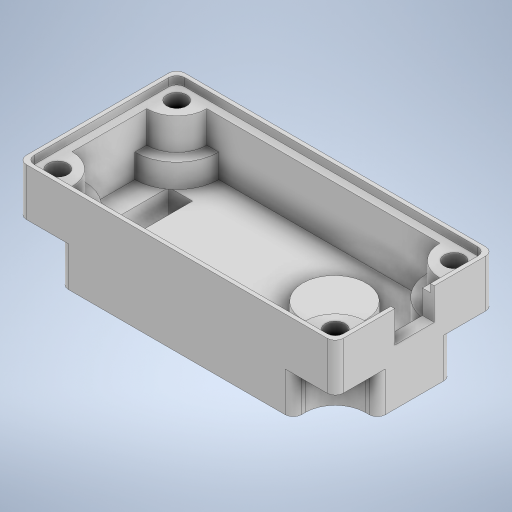
# Autodesk Inventor part: ServoCase
Saved by Autodesk Inventor 2024 (Build 280153000, 153)
## iProperties
Created: 2026-02-12
Part Number: ServoCase
Material: Generic
Document SubType Name: Modeling
Designer: Liam
Density: 1 g/cm^3
Appearance: Default
Author: Liam
Autodesk Inventor part; units mm, degrees
ref_plane "YZ Plane" through (0, 0, 0) normal (1, 0, 0) x (0, 1, 0)
ref_plane "XY Plane" through (0, 0, 0) normal (0, 0, 1) x (1, 0, 0)
sketch "Sketch1" plane through (0, 0, 0) normal (0, 1, 0) x (-1, 0, 0)
  line L0 (20, 10) -> (-20, 10)
  line L1 (-20, 10) -> (-20, -10)
  line L2 (-20, -10) -> (20, -10)
  line L3 (20, -10) -> (20, 10)
  line L4 (20, 10) -> (-20, -10) construction
  line L5 (-20, 10) -> (20, -10) construction
  line L6 (-18.5, 8.5) -> (18.5, 8.5)
  line L7 (18.5, 8.5) -> (18.5, -8.5)
  line L8 (18.5, -8.5) -> (-18.5, -8.5)
  line L9 (-18.5, -8.5) -> (-18.5, 8.5)
  circle A0 centre (17.5, 7.5) radius 1.25
  line L10 (0, 0) -> (18.5, 0) construction
  line L11 (0, 0) -> (0, 0.8088) construction
  line L12 (0, 0.8088) -> (0, 8.5) construction
  circle A1 centre (17.5, -7.5) radius 1.25
  circle A2 centre (-17.5, 7.5) radius 1.25
  circle A3 centre (-17.5, -7.5) radius 1.25
  line L13 (-19.5, 9.5) -> (19.5, 9.5)
  line L14 (19.5, 9.5) -> (19.5, -9.5)
  line L15 (19.5, -9.5) -> (-19.5, -9.5)
  line L16 (-19.5, -9.5) -> (-19.5, 9.5)
  arc A4 (14.7, 8.5) -> (18.5, 4.7) centre (18.5, 8.5) ccw
  arc A5 (18.5, -4.7) -> (14.7, -8.5) centre (18.5, -8.5) ccw
  arc A6 (-18.5, 4.7) -> (-14.7, 8.5) centre (-18.5, 8.5) ccw
  arc A7 (-14.7, -8.5) -> (-18.5, -4.7) centre (-18.5, -8.5) ccw
  arc A8 (18.5, -3.2) -> (13.2, -8.5) centre (18.5, -8.5) ccw
  arc A9 (13.2, 8.5) -> (18.5, 3.2) centre (18.5, 8.5) ccw
  arc A10 (-13.2, -8.5) -> (-18.5, -3.2) centre (-18.5, -8.5) ccw
  arc A11 (-18.5, 3.2) -> (-13.2, 8.5) centre (-18.5, 8.5) ccw
  line L17 (14.7, 8.5) -> (14.7, 10)
  line L18 (18.5, 4.7) -> (20, 4.7)
  line L19 (-14.7, 8.5) -> (-14.7, 10)
  line L20 (-18.5, 4.7) -> (-20, 4.7)
  line L21 (14.7, -8.5) -> (14.7, -10)
  line L22 (18.5, -4.7) -> (20, -4.7)
  line L23 (-18.5, -4.7) -> (-20, -4.7)
  line L24 (-14.7, -8.5) -> (-14.7, -10)
  point P0 (-14.7, -8.5)
  point P1 (-18.5, -4.7)
  point P2 (-18.5, 4.7)
  point P3 (-14.7, 8.5)
  point P4 (18.5, -4.7)
  point P5 (14.7, -8.5)
  point P6 (-13.2, -8.5)
  point P7 (-18.5, -3.2)
  point P8 (-18.5, 3.2)
  point P9 (-13.2, 8.5)
  point P10 (-18.5, -4.7)
  point P11 (-18.5, 4.7)
  point P12 (-20, 4.7)
  point P13 (-20, -4.7)
  point P14 (13.2, 8.5)
  point P15 (18.5, 3.2)
  point P16 (18.5, -3.2)
  point P17 (13.2, -8.5)
  point P18 (-14.7, -8.5)
  point P19 (-14.7, -10)
  point P20 (14.7, -10)
  point P21 (20, -4.7)
  point P22 (-14.7, 10)
  point P23 (-14.7, 8.5)
  dimension "d0" = 40
  dimension "d1" = 20
  dimension "d2" = 1.5
  dimension "d3" = 2.5
  dimension "d4" = 2.5
  dimension "d5" = 2.5
  dimension "d8" = 0.5
  dimension "d9" = 3.8
  dimension "d17" = 1.5
  constraints: 50 end point, 27 symmetric about line, 16 point on circle, 12 centre point, 6 parallel, 6 perpendicular, 4 midpoint, 4 point on line, 1 coincident, 1 horizontal, 15 other
  measures "d0" distance of L1.end L2.end
  measures "d1" distance of L0.end L1.end
  measures "d2" distance between parallel lines of L6 L0
  measures "d3" diameter of A0
  measures "d4" distance from line of L3 A0.centre
  measures "d5" distance from line of L0 A0.centre
  measures "d8" distance between parallel lines of L0 L13
  measures "d9" radius of A4
  measures "d17" radial gap between concentric circles of A8 A5
extrude "Extrusion1" add sketch "Sketch1" along normal blind 6 contours L3 L18 L14 L13 L17 L0 | L17 L13 L19 L0 | L3 L22 L14 L18 | L19 L13 L16 L20 L1 L0 | L3 L2 L21 L15 L14 L22 | L20 L16 L23 L1 | L2 L24 L15 L21 | L23 L16 L15 L24 L2 L1
extrude "Extrusion2" add sketch "Sketch1" along normal blind 5 contours L17 L6 L19 L13 | L13 L14 L18 L7 A0 L6 L17 | L14 L22 L7 L18 | L19 L6 A2 L9 L20 L16 L13 | L6 A0 L7 A4 | L14 L15 L21 L8 A1 L7 L22 | A6 L9 A2 L6 | L7 A1 L8 A5 | L20 L9 L23 L16 | L6 L7 A0 | L15 L24 L8 L21 | L23 L9 A3 L8 L24 L15 L16 | A2 L9 L6 | L7 L8 A1 | A7 L8 A3 L9 | A3 L8 L9 picked at (18.4219, 8.4219) picked at (-18.4219, 8.4219) picked at (18.4219, -8.4219) picked at (-18.4219, -8.4219)
sketch "Sketch2" plane through (0, 6, 0) normal (0, 1, 0) x (1, 0, 0)
  line L0 (-20, 10) -> (-20, -10) projected
  line L1 (-18.5, -4.7) -> (-18.5, 4.7) projected
  line L2 (-20, -2.5) -> (-18.5, -2.5)
  line L3 (-18.5, -2.5) -> (-18.5, 2.5)
  line L4 (-18.5, 2.5) -> (-20, 2.5)
  line L5 (-20, 2.5) -> (-20, -2.5)
  line L6 (0, 0) -> (0, 8.5) construction
  line L7 (-14.7, 8.5) -> (14.7, 8.5) construction
  line L8 (20, -2.5) -> (18.5, -2.5)
  line L9 (18.5, -2.5) -> (18.5, 2.5)
  line L10 (18.5, 2.5) -> (20, 2.5)
  line L11 (20, 2.5) -> (20, -2.5)
  point P0 (-20, 0)
  point P1 (-20, 2.5)
  point P2 (-18.5, -2.5)
  dimension "d12" = 1.5
  dimension "d13" = 5
  dimension "d14" = 2.5
  constraints: 18 end point, 4 symmetric about line, 2 midpoint, 2 parallel, 2 point on line, 1 horizontal, 1 perpendicular
  measures "d12" distance of L2.start L2.end
  measures "d13" distance between parallel lines of L4 L2
  measures "d14" distance from line of point (-20, 0) L2
extrude "Extrusion3" cut sketch "Sketch2" against normal blind 4 contours L8 L9 L10 L11
extrude "Extrusion5" add sketch "Sketch1" along normal blind 1 and the other way blind 5 contours L17 L13 L19 L0 | L3 L22 L14 L18 | L17 L6 L19 L13 | L14 L22 L7 L18 | A4 L7 A9 L6 | L20 L16 L23 L1 | L6 A11 L9 A6 | L2 L24 L15 L21 | A5 L8 A8 L7 | L20 L9 L23 L16 | L15 L24 L8 L21 | L9 A10 L8 A7
ref_plane "Work Plane1" through (0, -5, 0) normal (0, 1, 0) x (-1, 0, 0)
sketch "Sketch9" plane through (0, -5, 0) normal (0, 1, 0) x (-1, 0, 0)
  line L0 (-18.5, 4.7) -> (-20, 4.7) projected
  arc A0 (-14.7, -8.5) -> (-18.5, -4.7) centre (-18.5, -8.5) ccw projected
  line L1 (-20, 4.7) -> (-18.5, 4.7)
  line L2 (-18.5, 4.7) -> (-18.5, -4.7)
  line L3 (-18.5, -4.7) -> (-20, -4.7)
  line L4 (-20, -4.7) -> (-20, 4.7)
  line L5 (-14.7, -8.5) -> (-14.7, -10) projected
  line L6 (14.7, -10) -> (14.7, -8.5) projected
  line L7 (-14.7, -8.5) -> (14.7, -8.5)
  line L8 (14.7, -8.5) -> (14.7, -10)
  line L9 (14.7, -10) -> (-14.7, -10)
  line L10 (-14.7, -10) -> (-14.7, -8.5)
  line L11 (18.5, 4.7) -> (18.5, -4.7) projected
  line L12 (20, -10) -> (20, 10) projected
  line L13 (18.5, 4.7) -> (20, 4.7)
  line L14 (20, 4.7) -> (20, -4.7)
  line L15 (20, -4.7) -> (18.5, -4.7)
  line L16 (18.5, -4.7) -> (18.5, 4.7)
  line L17 (20, 10) -> (14.7, 10) projected
  line L18 (-14.7, 8.5) -> (-13.2, 8.5) projected
  line L19 (14.7, 10) -> (-14.7, 10)
  line L20 (-14.7, 10) -> (-14.7, 8.5)
  line L21 (-14.7, 8.5) -> (14.7, 8.5)
  line L22 (14.7, 8.5) -> (14.7, 10)
  arc A1 (-18.5, 4.7) -> (-14.7, 8.5) centre (-18.5, 8.5) ccw projected
  arc A2 (-18.5, 4.7) -> (-14.7, 8.5) centre (-18.5, 8.5) ccw
  arc A3 (-14.7, -8.5) -> (-18.5, -4.7) centre (-18.5, -8.5) ccw
  arc A4 (14.7, 8.5) -> (18.5, 4.7) centre (18.5, 8.5) ccw projected
  arc A5 (14.7, 8.5) -> (18.5, 4.7) centre (18.5, 8.5) ccw
  arc A6 (18.5, -4.7) -> (14.7, -8.5) centre (18.5, -8.5) ccw projected
  arc A7 (18.5, -4.7) -> (14.7, -8.5) centre (18.5, -8.5) ccw
  circle A8 centre (-9.9, 0) radius 2.5
  circle A9 centre (-9.9, 0) radius 4
  line L23 (-5.9, 3) -> (-3.9, 3)
  line L24 (-3.9, 3) -> (-3.9, -3)
  line L25 (-3.9, -3) -> (-5.9, -3)
  line L26 (-5.9, -3) -> (-5.9, 3)
  line L27 (-5.9, 3) -> (-3.9, -3) construction
  line L28 (-3.9, 3) -> (-5.9, -3) construction
  line L29 (-12.9, 4) -> (-12.9, 6)
  line L30 (-6.9, 4) -> (-12.9, 4)
  line L31 (-6.9, 6) -> (-6.9, 4)
  line L32 (-12.9, 6) -> (-6.9, 6)
  line L33 (-13.9, -3) -> (-15.9, -3)
  line L34 (-13.9, 3) -> (-13.9, -3)
  line L35 (-15.9, 3) -> (-13.9, 3)
  line L36 (-15.9, -3) -> (-15.9, 3)
  line L37 (-6.9, -4) -> (-6.9, -6)
  line L38 (-12.9, -4) -> (-6.9, -4)
  line L39 (-12.9, -6) -> (-12.9, -4)
  line L40 (-6.9, -6) -> (-12.9, -6)
  line L41 (12.5, -4.5) -> (15.5, -4.5)
  line L42 (15.5, -4.5) -> (15.5, 4.5)
  line L43 (15.5, 4.5) -> (12.5, 4.5)
  line L44 (12.5, 4.5) -> (12.5, -4.5)
  line L45 (12.5, -4.5) -> (15.5, 4.5) construction
  line L46 (15.5, -4.5) -> (12.5, 4.5) construction
  point P0 (0, 0)
  point P1 (18.5, 2.5)
  point P2 (20, -2.5)
  point P3 (18.5, 2.5)
  point P4 (-20, 0)
  point P5 (-4.9, 0)
  point P6 (14, 0)
  dimension "d58" = 5
  dimension "d59" = 10.1
  dimension "d60" = 0
  dimension "d62" = 2
  dimension "d63" = 6
  dimension "d64" = 0
  dimension "d65" = 5
  dimension "d68" = 360
  dimension "d80" = 3
  dimension "d81" = 9
  dimension "d82" = 6
  dimension "d83" = 10
  dimension "d87" = 8
  constraints: 80 end point, 12 parallel, 8 point on circle, 6 centre point, 6 horizontal, 6 perpendicular, 5 midpoint, 4 coincident, 2 point on line, 33 other
  measures "d58" diameter of A8
  measures "d59" distance from line of L4 A8.centre
  measures "d60" vertical distance of point (-20, 0) A8.centre
  measures "d62" distance of L24.end L25.end
  measures "d63" distance of L23.end L24.end
  measures "d64" vertical distance of point (0, 0) point (-4.9, 0)
  measures "d65" distance of A8.centre point (-4.9, 0)
  measures "d80" distance of L41.start L41.end
  measures "d81" distance of L41.end L42.end
  measures "d82" distance from line of L14 point (14, 0)
  measures "d83" distance from line of L19 point (14, 0)
  measures "d87" diameter of A9
extrude "Extrusion11" add sketch "Sketch9" along normal blind 3 contours A1 L18 L21 A4 L11 A6 L7 A0 L2 | L38 L37 L40 L39 | L34 L33 L36 L35 | L30 L29 L32 L31 | L26 L23 L24 L25 | L44 L43 L42 L41
extrude "Extrusion12" add sketch "Sketch9" along normal blind 5 contours A9
sketch "Sketch10" plane through (9.9, 0, 0) normal (0, 1, 0) x (1, 0, 0)
  circle A0 centre (0, 0) radius 4
  line L0 (8.6, -2.5) -> (8.6, 2.5) projected
  line L1 (4.8, -8.5) -> (-24.6, -8.5) projected
  point P0 (-9.9, 0)
  dimension "d72" = 8
  dimension "d73" = 8.6
  dimension "d74" = 8.5
  constraints: 1 centre point
  measures "d72" diameter of A0
  measures "d73" distance from line of L0 A0.centre
  measures "d74" distance from line of L1 A0.centre
extrude "Extrusion13" add sketch "Sketch10" along normal blind 0.5
extrude "Extrusion14" cut sketch "Sketch9" along normal blind 1.5 contours L38 L37 L40 L39 | L34 L33 L36 L35 | L30 L29 L32 L31 | L26 L23 L24 L25
fillet "Fillet5" radius 1 16 edges at (6.9, -4.25, -6) (6.9, -4.25, -4) (12.9, -4.25, -6) (12.9, -4.25, -4) (13.9, -4.25, -3) (15.9, -4.25, -3) (15.9, -4.25, 3) (13.9, -4.25, 3) (12.9, -4.25, 4) (12.9, -4.25, 6) (6.9, -4.25, 6) (6.9, -4.25, 4) (5.9, -4.25, 3) (3.9, -4.25, 3) (5.9, -4.25, -3) (3.9, -4.25, -3)
extrude "Extrusion15" cut sketch "Sketch9" along normal blind 3 contours L44 L43 L42 L41
fillet "Fillet6" radius 1 16 edges at (20, 3, -10) (20, 3, 10) (19.5, 5.5, -9.5) (19.5, 5.5, 9.5) (-20, 3, -10) (-19.5, 5.5, -9.5) (-20, 3, 10) (-19.5, 5.5, 9.5) (-20, -2.5, -4.7) (-20, -2.5, 4.7) (-14.7, -2.5, -10) (-14.7, -2.5, 10) (14.7, -2.5, -10) (20, -2.5, -4.7) (20, -2.5, 4.7) (14.7, -2.5, 10)
equation "\"d0\" = CaseLength"
equation "\"d1\" = CaseWidth"
equation "\"d3\" = ScrewDiameter"
equation "\"d4\" = ScrewDis"
equation "\"d5\" = ScrewDis"
equation "\"CaseWidth\" = 20"
equation "\"CaseLength\" = 40"
equation "\"CaseThickness\" = 2"
equation "\"CaseScrewHeight\" = 5"
equation "\"ScrewDiameter\" = 2.5"
equation "\"ScrewDis\" = 2.5"
equation "\"FloorDiff\" = 5"
equation "\"FloorHeight\" = 3"
body "Solid1"
